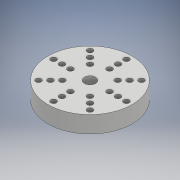
# Autodesk Inventor part: Hand Polley v2
Saved by Autodesk Inventor 2018 (Build 220112000, 112)
## iProperties
Created: 2018-04-10
Part Number: Hand Polley v2
Material: Générique
Document SubType Name: Modeling
Designer: Thomas
Density: 1 g/cm^3
Appearance: Par défaut
Author: Thomas
Autodesk Inventor part; units mm, degrees
ref_plane "YZ Plane" through (0, 0, 0) normal (1, 0, 0) x (0, 1, 0)
ref_plane "XZ Plane" through (0, 0, 0) normal (0, 1, 0) x (-1, 0, 0)
ref_plane "XY Plane" through (0, 0, 0) normal (0, 0, 1) x (1, 0, 0)
sketch "Esquisse1" plane through (0, 0, 0) normal (0, 0, 1) x (1, 0, 0)
  circle A0 centre (0, 0) radius 15
  circle A1 centre (0, 0) radius 2
  dimension "d0" = 4
  dimension "d1" = 30
  constraints: 2 centre point, 2 coincident
  measures "d0" diameter of A1
  measures "d1" diameter of A0
extrude "Extrusion1" add sketch "Esquisse1" along normal blind 6
sketch "Esquisse2" plane through (0, 0, 6) normal (0, 0, 1) x (1, 0, 0)
  circle A0 centre (0, 0) radius 15 construction
  line L0 (-15, 0) -> (15, 0) construction
  line L1 (-10.603, 10.6102) -> (10.603, -10.6102) construction
  circle A1 centre (-7.0687, 7.0734) radius 1
  circle A2 centre (-4.9481, 4.9514) radius 1
  circle A3 centre (-9.1893, 9.1955) radius 1
  line L2 (-10.603, -10.6102) -> (10.603, 10.6102) construction
  line L3 (0, 15) -> (0, -15) construction
  circle A4 centre (0, 0) radius 13 construction
  circle A5 centre (0, 0) radius 10 construction
  circle A6 centre (0, 0) radius 7 construction
  circle A7 centre (-13, 0.0044) radius 1
  circle A8 centre (-10, 0.0034) radius 1
  circle A9 centre (-7, 0.0024) radius 1
  circle A10 centre (-9.1955, -9.1893) radius 1
  circle A11 centre (-7.0734, -7.0687) radius 1
  circle A12 centre (-4.9514, -4.9481) radius 1
  circle A13 centre (-0.0044, -13) radius 1
  circle A14 centre (-0.0034, -10) radius 1
  circle A15 centre (-0.0024, -7) radius 1
  circle A16 centre (9.1893, -9.1955) radius 1
  circle A17 centre (7.0687, -7.0734) radius 1
  circle A18 centre (4.9481, -4.9514) radius 1
  circle A19 centre (13, -0.0044) radius 1
  circle A20 centre (10, -0.0034) radius 1
  circle A21 centre (7, -0.0024) radius 1
  circle A22 centre (9.1955, 9.1893) radius 1
  circle A23 centre (7.0734, 7.0687) radius 1
  circle A24 centre (4.9514, 4.9481) radius 1
  circle A25 centre (0.0044, 13) radius 1
  circle A26 centre (0.0034, 10) radius 1
  circle A27 centre (0.0024, 7) radius 1
  point P0 (-1.4132, 1.4141)
  dimension "d42" = 2
  dimension "d43" = 2
  dimension "d44" = 2
  dimension "d48" = 3
  dimension "d49" = 2
  dimension "d50" = 3
  dimension "d60" = 360
  constraints: 24 centre point, 8 end point, 4 point on line, 3 coincident, 1 horizontal, 1 vertical, 67 other
  measures "d42" diameter of A3
  measures "d43" diameter of A1
  measures "d44" diameter of A2
  measures "d48" distance of A1.centre A3.centre
  measures "d49" distance of L1.start A3.centre
  measures "d50" distance of A2.centre A1.centre
extrude "Extrusion3" cut sketch "Esquisse2" against normal blind 6
